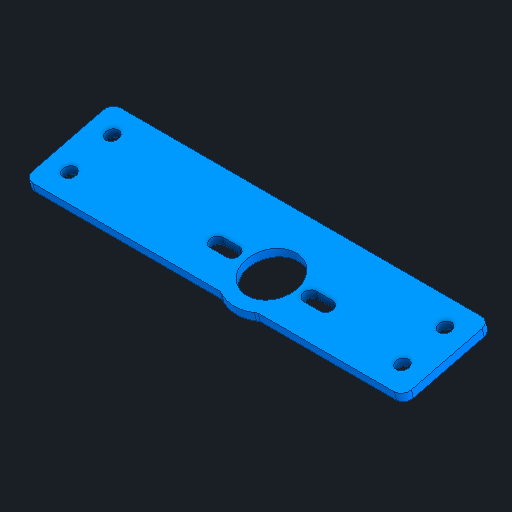
# Autodesk Inventor part: motor_mount_plate
Saved by Autodesk Inventor 2023 (Build 270158030, 158C)
## iProperties
Created: 2022-03-30
Part Number: motor_mount_plate
Material: Generic
Document SubType Name: Modeling
Designer: kardo
Density: 1 g/cm^3
Appearance: Blue Plastic
Author: kardo
Autodesk Inventor part; units mm, degrees
ref_plane "YZ Plane" through (0, 0, 0) normal (1, 0, 0) x (0, 1, 0)
ref_plane "XZ Plane" through (0, 0, 0) normal (0, 1, 0) x (-1, 0, 0)
ref_plane "XY Plane" through (0, 0, 0) normal (0, 0, 1) x (1, 0, 0)
derived "stencil_frame.ipt"
sketch "sk_cowl_joint_locations" plane through (54.6, 0, 0) normal (1, 0, 0) x (0, 1, 0)
  line L0 (-363, 18.496) -> (-275.8801, 19.4795) construction
  arc A0 (-275.8801, 19.4795) -> (-254.1001, 19.9549) centre (-287.5515, 1053.3708) ccw construction
  line L1 (-254.1001, 19.9549) -> (9.48, 28.4869) construction
  arc A1 (30.81, 28.832) -> (9.48, 28.4869) centre (30.81, -630.4631) ccw construction
  line L2 (30.81, 28.832) -> (94.8, 28.832) construction
  line L3 (94.8, 30.032) -> (30.81, 30.032) construction
  arc A2 (30.81, 30.032) -> (9.4412, 29.6862) centre (30.81, -630.4631) ccw construction
  line L4 (9.4412, 29.6862) -> (-254.1389, 21.1542) construction
  arc A3 (-275.8936, 20.6794) -> (-254.1389, 21.1542) centre (-287.5515, 1053.3708) ccw construction
  line L5 (-275.8936, 20.6794) -> (-363, 19.6961) construction
  line L6 (-242.0001, 1541.8302) -> (-242.0001, -1877.3857) construction
  line L7 (-120.9999, 1541.8302) -> (-120.9999, -1877.3857) construction
  line L8 (-363, 1541.8302) -> (-363, -1877.3857) construction
  line L9 (0, 1541.8302) -> (0, -1877.3857) construction
  line L10 (-242.0001, 45.0688) -> (-242.0001, 21.5472) construction
  line L11 (-120.9999, 49.9661) -> (-120.9999, 25.4639) construction
  line L12 (-363, 19.6961) -> (-363, 19.6961)
  line L13 (-363, 19.6961) -> (-363, 36.9211) construction
  line L14 (-513.5712, 1550.2518) -> (344.0815, -1889.6051) construction
  line L15 (-362.7741, 36.9211) -> (-363, 39.712) construction
  line L16 (0, 51.6) -> (0, 29.3806) construction
  line L17 (-142.5135, 45.4866) -> (-137.389, 24.9334) construction
  line L18 (-134.789, 31.0394) -> (-138.6702, 30.0717) construction
  line L19 (-137.3512, 41.316) -> (-141.2324, 40.3483) construction
  line L20 (-142.5135, 45.4866) -> (-138.6324, 46.4543) construction
  line L21 (-137.389, 24.9334) -> (-133.5079, 25.9011) construction
  line L22 (-138.6324, 46.4543) -> (-138.8117, 52.2515) construction
  spline S0 degree 2 poles (-363, 39.712) (-181.6483, 54.394) (0, 54.4) knots 0 0 0 1 1 1
  spline S1 degree 3 poles (0, 54.4) (52.14, 54.4) (75.84, 49.3408) (94.8, 37.536) knots 1 1 1 1 2 2 2 2
  spline S2 degree 3 poles (93.3201, 35.1591) (91.7887, 36.1125) (88.6673, 37.9255) (84.5441, 39.9679) (80.1975, 41.8496) (76.5188, 43.2287) (71.6118, 44.7991) (67.4172, 45.9339) (61.7832, 47.203) (56.9422, 48.0997) (50.4217, 49.0741) (44.8094, 49.7373) (37.2484, 50.4231) (30.743, 50.8582) (21.9903, 51.263) (12.5916, 51.53) (4.3299, 51.6) (0, 51.6) knots 1 1 1 1 1.083333 1.166667 1.208333 1.291667 1.333333 1.416667 1.458333 1.541667 1.583333 1.666667 1.708333 1.791667 1.833333 1.916667 2 2 2 2
  spline S3 degree 3 poles (0, 51.6) (-20.1706, 51.5993) (-55.4643, 51.3605) (-95.7903, 50.6123) (-126.0307, 49.8474) (-146.1889, 49.2356) (-171.3841, 48.3435) (-191.5382, 47.528) (-216.7283, 46.3813) (-236.8783, 45.3621) (-262.0632, 43.9608) (-282.2091, 42.7379) (-307.3889, 41.082) (-332.5661, 39.2987) (-352.7052, 37.7363) (-362.7741, 36.9211) knots 0 0 0 0 0.166667 0.291667 0.333333 0.416667 0.458333 0.541667 0.583333 0.666666 0.708333 0.791666 0.833333 0.916666 1 1 1 1
  point P0 (0, 0)
  point P1 (-363, 28.3086)
  point P2 (-242.0001, 33.308)
  point P3 (-120.9999, 37.715)
  point P4 (0, 40.4903)
  point P5 (0, 40.4903)
ref_plane "plane_motor_mount" through (0, -127.05, 0) normal (0, 0.9702957, 0.2419219) x (-1, 0, 0)
ref_plane "plane_symmetry" through (0, 0, 0) normal (1, 0, 0) x (0, 1, 0)
sketch "sk_drivetrain_profile" plane through (6, 0, 0) normal (1, 0, 0) x (0, 1, 0)
  line L0 (-547.3485, 0) -> (393.091, 0) construction
  line L1 (-363, 1541.8302) -> (-363, -1877.3857) construction
  line L2 (0, 1541.8302) -> (0, -1877.3857) construction
  line L3 (-140.12, 52.421) -> (-133.3462, 25.2528)
  line L4 (-388, 0) -> (-343.0839, 2.7472)
  line L5 (-136.7331, 38.8369) -> (-223.8252, 17.1224)
  line L6 (-300.1691, 5.372) -> (-261.4573, 7.7397) construction
  line L7 (-261.4573, 7.7397) -> (-223.8252, 17.1224) construction
  line L8 (-133.3462, 25.2528) -> (-133.3462, 20.2528) construction
  line L9 (-343.0839, 2.7472) -> (-300.1691, 5.372)
  line L10 (-513.5712, 1550.2518) -> (344.0815, -1889.6051) construction
  line L11 (-224.4013, 19.4329) -> (-137.3092, 41.1474) construction
  line L12 (-136.1571, 36.5264) -> (-223.2491, 14.8119) construction
  line L13 (-224.4013, 19.4329) -> (-223.2491, 14.8119) construction
  spline S0 degree 2 poles (-300.1691, 5.372) (-261.4573, 7.7397) (-223.8252, 17.1224) knots 1 1 1 2 2 2
  line L14 (0, 18.496) -> (-254.1001, 19.5569) construction
  line L15 (-55.187, 19.9264) -> (-309.3336, 20.9876) construction
  point P0 (0, 0)
  point P1 (-214.7203, 19.3925)
  point P2 (-205.0394, 19.3521)
  point P3 (-200.3057, 20.5323)
derived "parameters_frame.ipt"
sketch "sk_base" plane through (0, -127.05, 0) normal (0, 0.9702957, 0.2419219) x (-1, 0, 0)
  line L0 (0, -1016.1573) -> (0, 1435.4387) projected
  line L1 (-44.6, 47.8764) -> (-44.6, 26.694)
  line L2 (-44.6, 26.694) -> (0, 26.694)
  line L3 (-44.6, 47.8764) -> (0, 47.8764)
  point P0 (0, -30.7362)
  point P1 (-54.6, 47.8764)
  point P2 (-54.6, 26.694)
  dimension "d1" = 10
  constraints: 6 end point, 4 point on line, 2 perpendicular, 1 parallel
  measures "d1" distance from line of point (-54.6, 47.876) L1
extrude "base" add sketch "sk_base" against normal blind 2
sketch "sk_drill_joint" plane through (0, -127.05, 0) normal (0, 0.9702957, 0.2419219) x (-1, 0, 0)
  line L0 (-44.6, 47.8764) -> (-44.6, 26.694) construction
  line L1 (-44.6, 47.8764) -> (0, 47.8764) construction
  line L2 (-44.6, 26.694) -> (0, 26.694) construction
  circle A0 centre (-39.2, 32.094) radius 1.5
  circle A1 centre (-39.2, 42.4764) radius 1.5
  line L3 (-39.2, 42.4764) -> (-39.2, 47.8764) construction
  line L4 (-39.2, 42.4764) -> (-39.2, 32.094) construction
  line L5 (-39.2, 32.094) -> (-39.2, 26.694) construction
  line L6 (-39.2, 42.4764) -> (-44.6, 42.4764) construction
  line L7 (-39.2, 32.094) -> (-44.6, 32.094) construction
  point P0 (0, -30.7362)
  dimension "d3" = 3
  dimension "d4" = 5.4
  constraints: 10 end point, 4 perpendicular, 4 point on line, 2 centre point, 2 collinear, 1 coincident, 1 equal radius, 1 parallel
  measures "d3" diameter of A1
  measures "d4" distance between parallel lines of L0 L4
extrude "drill_joint" cut sketch "sk_drill_joint" along normal through all both and the other way through all
mirror "mirror" about plane through (0, 0, 0) normal (1, 0, 0)
sketch "sk_expand_motor" plane through (0, -127.05, 0) normal (0, 0.9702957, 0.2419219) x (-1, 0, 0)
  line L0 (-6, 54.0258) -> (-6, 26.0258) construction
  line L1 (-9.8571, 48.1574) -> (-21.2857, 42.7364)
  arc A0 (-21.2857, 42.7364) -> (-21.2857, 37.3153) centre (-20, 40.0258) ccw
  line L2 (-21.2857, 37.3153) -> (-9.8571, 31.8943)
  arc A1 (-9.8571, 31.8943) -> (-2.1429, 31.8943) centre (-6, 40.0258) ccw
  line L3 (-2.1429, 31.8943) -> (9.2857, 37.3153)
  arc A2 (9.2857, 37.3153) -> (9.2857, 42.7364) centre (8, 40.0258) ccw
  line L4 (9.2857, 42.7364) -> (-2.1429, 48.1574)
  arc A3 (-2.1429, 48.1574) -> (-9.8571, 48.1574) centre (-6, 40.0258) ccw
  line L5 (-20, 40.0258) -> (8, 40.0258) construction
  point P0 (0, -30.7362)
  dimension "d23" = 28
  dimension "d24" = 18
  dimension "d26" = 6
  constraints: 10 end point, 8 point on circle, 8 tangent, 4 centre point, 3 midpoint, 2 coincident, 2 equal radius, 1 perpendicular
  measures "d23" distance of L5.end L5.start
  measures "d24" diameter of A3
  measures "d26" diameter of A2
extrude "expand_motor" add sketch "sk_expand_motor" against normal blind 2
sketch "sk_drill_motor" plane through (0, -127.05, 0) normal (0, 0.9702957, 0.2419219) x (-1, 0, 0)
  circle A0 centre (-6, 40.0258) radius 6
  line L0 (-15, 40.0258) -> (-19, 40.0258) construction
  line L1 (-15, 41.5258) -> (-19, 41.5258)
  line L2 (-19, 38.5258) -> (-15, 38.5258)
  arc A1 (-15, 38.5258) -> (-15, 41.5258) centre (-15, 40.0258) ccw
  arc A2 (-19, 41.5258) -> (-19, 38.5258) centre (-19, 40.0258) ccw
  line L3 (3, 40.0258) -> (7, 40.0258) construction
  line L4 (3, 38.5258) -> (7, 38.5258)
  line L5 (7, 41.5258) -> (3, 41.5258)
  arc A3 (3, 41.5258) -> (3, 38.5258) centre (3, 40.0258) ccw
  arc A4 (7, 38.5258) -> (7, 41.5258) centre (7, 40.0258) ccw
  line L6 (-15, 40.0258) -> (-6, 40.0258) construction
  line L7 (-6, 40.0258) -> (3, 40.0258) construction
  line L8 (-6, 54.0258) -> (-6, 26.0258) construction
  point P0 (0, -30.7362)
  point P1 (-17, 40.0258)
  point P2 (5, 40.0258)
  dimension "d9" = 12
  dimension "d14" = 3
  dimension "d15" = 4
  dimension "d21" = 18
  constraints: 20 end point, 8 point on circle, 8 tangent, 5 centre point, 5 collinear, 2 midpoint, 2 parallel, 1 equal radius, 1 perpendicular
  measures "d9" diameter of A0
  measures "d14" diameter of A2
  measures "d15" distance of L2.start L2.end
  measures "d21" distance of L3.start L0.start
extrude "drill_motor" cut sketch "sk_drill_motor" along normal through all both and the other way through all
fillet "round_corners" radius 2 4 edges at (44.6, -139.6026, 46.2123) (44.6, -134.4782, 25.6592) (-44.6, -139.6026, 46.2123) (-44.6, -134.4782, 25.6592)
derived "parameters_powertrain.ipt"
equation "\"d1\" = cowl_sealing_width + cowl_liner_width"
equation "\"d3\" = drill_motor_mount_diam"
equation "\"d4\" = 1.8 * drill_motor_mount_diam"
equation "\"d27\" = bulkhead_thickness"
equation "\"d18\" = 0.5 * bulkhead_inset"
equation "\"drill_motor_mount_diam\" = 3"
equation "\"bulkhead_thickness\" = 2"
equation "\"bulkhead_inset\" = 4"
equation "\"cowl_sealing_width\" = 5"
equation "\"cowl_liner_width\" = 5"
body "Solid1"
